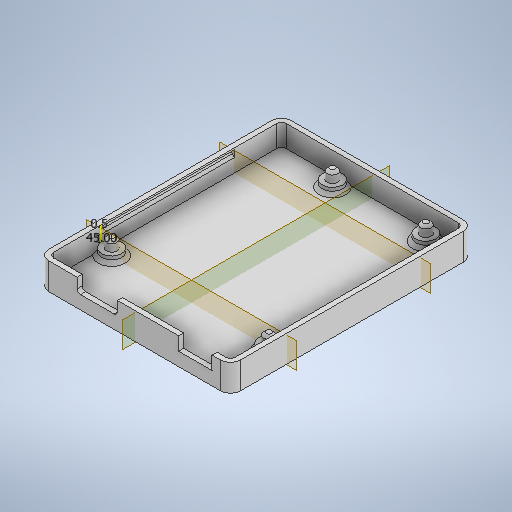
# Autodesk Inventor part: uno_r4_base
Saved by Autodesk Inventor 2025.2 (Build 292293000, 293)
## iProperties
Created: 2025-03-24
Part Number: uno_r4_base
Material: Generic
Document SubType Name: Modeling
Designer: caomi
Density: 1 g/cm^3
Appearance: Default
Author: caomi
Autodesk Inventor part; units mm, degrees
ref_plane "YZ Plane" through (0, 0, 0) normal (1, 0, 0) x (0, 1, 0)
ref_plane "XZ Plane" through (0, 0, 0) normal (0, 1, 0) x (-1, 0, 0)
sketch "Sketch1" plane through (0, 0, 0) normal (0, 1, 0) x (-1, 0, 0)
  line L0 (0, 0) -> (53.34, 0) construction
  line L1 (53.34, 0) -> (53.34, -68.58) construction
  line L2 (53.34, -68.58) -> (0, -68.58) construction
  line L3 (0, -68.58) -> (0, 0) construction
  line L4 (55.34, -70.58) -> (55.34, 2)
  line L5 (55.34, 2) -> (-2, 2)
  line L6 (-2, 2) -> (-2, -70.58)
  line L7 (-2, -70.58) -> (55.34, -70.58)
  dimension "d0" = 53.34
  dimension "d1" = 68.58
  dimension "d2" = 2
  constraints: 16 end point, 4 parallel, 2 perpendicular, 1 horizontal, 3 other
  measures "d0" distance of L0.start L0.end
  measures "d1" distance of L2.end L0.start
  measures "d2" distance between parallel lines of L1 L4
extrude "Extrusion1" add sketch "Sketch1" along normal blind 8
fillet "Fillet2" radius 3 4 edges at (-55.34, 4, 2) (-55.34, 4, -70.58) (2, 4, -70.58) (2, 4, 2)
shell "Shell1" thickness 1.5 removed faces 1 at (-17.1133, 8, -45.3867)
sketch "Sketch2" plane through (0, 8, 0) normal (0, 1, 0) x (1, 0, 0)
  line L0 (-1, -0.5) -> (-52.34, -0.5) projected
  line L1 (-55.34, -2) -> (2, -2) projected
  line L2 (-43.84, -0.5) -> (-31.84, -0.5)
  line L3 (-31.84, -0.5) -> (-31.84, -2)
  line L4 (-31.84, -2) -> (-43.84, -2)
  line L5 (-43.84, -2) -> (-43.84, -0.5)
  line L6 (-13.54, -0.5) -> (-3.54, -0.5)
  line L7 (-3.54, -0.5) -> (-3.54, -2)
  line L8 (-3.54, -2) -> (-13.54, -2)
  line L9 (-13.54, -2) -> (-13.54, -0.5)
  line L10 (-53.34, 0) -> (-53.34, 68.58) construction
  point P0 (-53.84, -0.5)
  point P1 (-53.84, 69.08)
  point P2 (0.5, 69.08)
  point P3 (0.5, -0.5)
  point P4 (0, 0)
  point P5 (-31.84, -0.5)
  point P6 (-13.54, -2)
  point P7 (-3.54, -0.5)
  point P8 (-53.84, 0.1213)
  point P9 (-53.84, 68.4587)
  point P10 (-53.2187, 69.08)
  point P11 (-0.1213, 69.08)
  point P12 (0.5, 68.4587)
  point P13 (0.5, 0.1213)
  point P14 (-0.1213, -0.5)
  point P15 (-53.2187, -0.5)
  dimension "d25" = 12
  dimension "d26" = 10
  dimension "d27" = 9.5
  dimension "d28" = 39.8
  constraints: 16 end point, 4 parallel, 4 point on line, 2 horizontal, 2 perpendicular
  measures "d25" distance of L3.end L4.end
  measures "d26" distance of L7.end L8.end
  measures "d27" horizontal distance of L10.start L4.end
  measures "d28" horizontal distance of L8.end L10.start
extrude "Extrusion2" cut sketch "Sketch2" against normal blind 4 contours L7 L1 L9 L0 | L3 L1 L5 L0
sketch "Sketch3" plane through (-53.84, 1.5, -69.08) normal (0, 1, 0) x (1, 0, 0)
  line L0 (53.84, -69.08) -> (0.5, -69.08) construction
  line L1 (0.5, -69.08) -> (0.5, -0.5) construction
  line L2 (53.84, -0.5) -> (53.84, -69.08) construction
  line L3 (0.5, -0.5) -> (53.84, -0.5) construction
  circle A0 centre (3.04, -53.84) radius 1.6
  circle A1 centre (51.3, -55.11) radius 1.6
  circle A2 centre (18.28, -3.04) radius 1.6
  circle A3 centre (46.22, -3.04) radius 1.6
  circle A4 centre (3.04, -53.84) radius 3
  circle A5 centre (51.3, -55.11) radius 3
  circle A6 centre (46.22, -3.04) radius 3
  circle A7 centre (18.28, -3.04) radius 3
  dimension "d12" = 15.24
  dimension "d13" = 2.54
  dimension "d14" = 13.97
  dimension "d15" = 50.8
  dimension "d16" = 66.04
  dimension "d17" = 17.78
  dimension "d18" = 45.72
  dimension "d19" = 3.2
  dimension "d20" = 6
  constraints: 8 centre point, 6 equal radius, 4 coincident, 1 horizontal alignment
  measures "d12" distance from line of L0 A0.centre
  measures "d13" distance from line of L1 A0.centre
  measures "d14" distance from line of L0 A1.centre
  measures "d15" distance from line of A1.centre L1
  measures "d16" distance from line of A2.centre L0
  measures "d17" distance from line of A2.centre L1
  measures "d18" horizontal distance of L0.end A3.centre
  measures "d19" diameter of A0
  measures "d20" diameter of A4
fillet "Fillet3" radius 1 2 edges at (-43.84, 4, 1.25) (-31.84, 4, 1.25)
extrude "Extrusion3" add sketch "Sketch3" along normal blind 5 contours A0 | A1 | A2 | A3
extrude "Extrusion4" add sketch "Sketch3" along normal blind 2
chamfer "Chamfer1" distance 1 angle 45 4 edges at (-53.8, 1.5, -15.24) (-38.56, 1.5, -66.04) (-10.62, 1.5, -66.04) (-5.54, 1.5, -13.97)
chamfer "Chamfer2" distance 0.8 angle 45 4 edges at (-52.4, 6.5, -15.24) (-37.16, 6.5, -66.04) (-9.22, 6.5, -66.04) (-4.14, 6.5, -13.97)
ref_plane "Work Plane1" through (0, 0, -15) normal (0, 0, 1) x (1, 0, 0)
ref_plane "Work Plane2" through (0, 0, -55) normal (0, 0, 1) x (1, 0, 0)
sketch "Sketch4" plane through (0, 0, -15) normal (0, 0, 1) x (1, 0, 0)
  line L0 (-53.84, 1.5) -> (-53.84, 8) projected
  line L1 (-53.84, 7.5) -> (-54.84, 6.5)
  line L2 (-54.84, 6.5) -> (-53.84, 5.5)
  line L3 (-54.84, 6.5) -> (-53.84, 6.5) construction
  point P0 (0, 0)
  dimension "d48" = 45
  dimension "d49" = 1
  dimension "d50" = 0.5
  constraints: 6 end point, 3 point on line, 2 perpendicular
  measures "d48" angle of L0 L2
  measures "d49" distance from line of L0 L1.end
  measures "d50" distance of L0.end L1.start
ref_plane "Work Plane3" through (-26.67, 0, -67.58) normal (-1, 0, 0) x (0, 0, 1)
extrude "Extrusion6" cut sketch "Sketch4" against normal up to surface (40 mm away)
fillet "Fillet4" radius 0.5 1 edges at (-54.84, 6.5, -35)
mirror "Mirror2" about plane through (-26.67, 0, -67.58) normal (-1, 0, 0) of "Extrusion6", "Fillet4"
body "Solid1"
